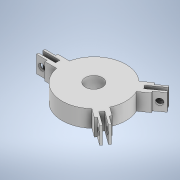
# Autodesk Inventor part: actuatorLink
Saved by Autodesk Inventor 2021 (Build 250183000, 183)
## iProperties
Created: 2020-12-19
Part Number: actuatorLink
Material: Generic
Document SubType Name: Modeling
Designer: awitc
Density: 1 g/cm^3
Appearance: Default
Author: awitc
Autodesk Inventor part; units mm, degrees
ref_plane "YZ Plane" through (0, 0, 0) normal (1, 0, 0) x (0, 1, 0)
ref_plane "XZ Plane" through (0, 0, 0) normal (0, 1, 0) x (-1, 0, 0)
ref_plane "XY Plane" through (0, 0, 0) normal (0, 0, 1) x (1, 0, 0)
sketch "Sketch1" plane through (0, 0, 0) normal (0, 1, 0) x (-1, 0, 0)
  circle A0 centre (-0.1978, 0.0875) radius 15
  line L0 (0, 0) -> (25, 0)
  line L1 (0, 0) -> (-20.2254, -14.6946)
  line L2 (0, 0) -> (25, 0) construction
  line L3 (0, 0) -> (-20.2254, 14.6946)
  line L4 (0, 0) -> (25, 0) construction
  line L5 (25, 0) -> (14.5167, 0)
  line L6 (25, 0) -> (14.481, 0)
  line L7 (25, 2) -> (20, 2)
  line L8 (20, 2) -> (20, -2)
  line L9 (20, -2) -> (25, -2)
  line L10 (20, -2) -> (20, -3)
  line L11 (20, 2) -> (20, 3)
  line L12 (25, -2) -> (25, 2)
  line L13 (20, 3) -> (14.5167, 3)
  line L14 (20, -3) -> (14.481, -3)
  line L15 (-21.401, 13.0766) -> (-17.3559, 10.1377)
  line L16 (-17.3559, 10.1377) -> (-17.9437, 9.3287)
  line L17 (-19.0499, 16.3127) -> (-15.0048, 13.3737)
  line L18 (-15.0048, 13.3737) -> (-14.417, 14.1828)
  line L19 (-19.0499, 16.3127) -> (-21.401, 13.0766)
  line L20 (-17.9437, 9.3287) -> (-13.832, 6.3413)
  line L21 (-14.417, 14.1828) -> (-10.2902, 11.1845)
  line L22 (-19.0499, -16.3127) -> (-15.0048, -13.3737)
  line L23 (-15.0048, -13.3737) -> (-14.417, -14.1828)
  line L24 (-17.9437, -9.3287) -> (-17.3559, -10.1377)
  line L25 (-17.3559, -10.1377) -> (-21.401, -13.0766)
  line L26 (-19.0499, -16.3127) -> (-21.401, -13.0766)
  line L27 (-14.417, -14.1828) -> (-10.1826, -11.1063)
  line L28 (-17.9437, -9.3287) -> (-13.7712, -6.2971)
  line L29 (-17.9437, -9.3287) -> (-12.7862, -9.3287) construction
  point P0 (22.9129, 10)
  point P1 (-9.5074, 11.849)
  point P2 (-14.229, 5.3909)
  point P3 (-14.2604, -5.1319)
  point P4 (-9.5775, -11.6181)
  point P5 (14.2709, 4.0444)
  point P6 (14.247, -3.9556)
  dimension "d87" = 25
  dimension "d88" = 25
  dimension "d89" = 144
  dimension "d90" = 25
  dimension "d91" = 144
  dimension "d146" = 5
  dimension "d147" = 4
  dimension "d149" = 5
  dimension "d151" = 5
  dimension "d153" = 5
  dimension "d154" = 1
  dimension "d155" = 36
  constraints: 60 end point, 5 horizontal, 4 perpendicular, 3 equal length, 2 parallel, 2 point on line, 1 vertical, 14 other
  measures "d87" distance of L0.start L0.end
  measures "d88" distance of L0.start L1.end
  measures "d89" angle of L1 L2
  measures "d90" distance of L0.start L3.end
  measures "d91" angle of L4 L3
  measures "d146" distance of L7.start L7.end
  measures "d147" distance of L7.end L8.end
  measures "d149" distance of L15.start L15.end
  measures "d151" distance of L17.start L17.end
  measures "d153" distance of L22.start L22.end
  measures "d154" distance of L24.start L24.end
  measures "d155" angle of L29 L28
extrude "Extrusion1" add sketch "Sketch1" along normal blind 8
sketch "Sketch8" plane through (0, 8, 0) normal (0, 1, 0) x (1, 0, 0)
  circle A0 centre (0, 0) radius 4
  dimension "d80" = 8
  constraints: 1 centre point
  measures "d80" diameter of A0
extrude "Extrusion8" cut sketch "Sketch8" against normal blind 10
sketch "Sketch28" plane through (19.0499, 0, -16.3127) normal (0.809, 0, -0.5878) x (-0.5878, 0, -0.809)
  line L0 (-4, 8) -> (0, 8) projected
  line L1 (-2, 8) -> (-2, 0)
  line L2 (-2, 0) -> (-1, 0)
  line L3 (-4, 0) -> (0, 0) projected
  line L4 (-1, 0) -> (-1, 8)
  line L5 (-1, 8) -> (-3, 8)
  line L6 (-3, 8) -> (-3, 0)
  line L7 (-3, 0) -> (-1, 0)
  point P0 (-3, 8)
  point P1 (-3, 0)
  point P2 (-1, 8)
  dimension "d156" = 1
  dimension "d157" = 2
  constraints: 12 end point, 3 perpendicular, 2 point on line, 1 collinear, 1 midpoint, 1 vertical
  measures "d156" distance of L1.end L2.end
  measures "d157" distance of L4.end L5.end
extrude "Extrusion26" cut sketch "Sketch28" against normal blind 8
sketch "Sketch29" plane through (21.401, 0, 13.0766) normal (0.809, 0, 0.5878) x (0.5878, 0, -0.809)
  line L0 (-4, 8) -> (0, 8) projected
  line L1 (-2, 0) -> (-1, 0)
  line L2 (-1, 0) -> (-1, 8)
  line L3 (-1, 8) -> (-2, 8)
  line L4 (-2, 8) -> (-2, 0)
  line L5 (-4, 0) -> (0, 0) projected
  line L6 (-1, 8) -> (-3, 8)
  line L7 (-3, 8) -> (-3, 0)
  line L8 (-3, 0) -> (-1, 0)
  line L9 (-1, 0) -> (-1, 8)
  point P0 (-3, 8)
  dimension "d160" = 1
  dimension "d161" = 2
  constraints: 16 end point, 4 parallel, 2 horizontal, 2 perpendicular, 2 point on line
  measures "d160" distance of L3.end L2.end
  measures "d161" distance of L8.end L7.end
extrude "Extrusion27" cut sketch "Sketch29" against normal blind 8
sketch "Sketch30" plane through (-25, 0, -2) normal (-1, 0, 0) x (0, 0, 1)
  line L0 (8.3413, 8) -> (-4.2971, 8) projected
  line L1 (2, 0) -> (3, 0)
  line L2 (3, 0) -> (3, 8)
  line L3 (3, 8) -> (2, 8)
  line L4 (2, 8) -> (2, 0)
  line L5 (8.3413, 0) -> (-4.2971, 0) projected
  line L6 (2, 8) -> (1, 8)
  line L7 (1, 8) -> (1, 0)
  line L8 (1, 0) -> (2, 0)
  line L9 (2, 0) -> (2, 8)
  dimension "d164" = 1
  dimension "d165" = 1
  constraints: 16 end point, 4 parallel, 2 horizontal, 2 perpendicular, 2 point on line
  measures "d164" distance of L3.end L2.end
  measures "d165" distance of L8.end L7.end
extrude "Extrusion28" cut sketch "Sketch30" against normal blind 8
sketch "Sketch31" plane through (-25, 0, 2) normal (0, 0, 1) x (1, 0, 0)
  line L0 (5, 8) -> (0, 8) projected
  line L1 (0, 8) -> (4.994, 0)
  line L2 (0, 0) -> (8, 0) projected
  circle A0 centre (2.497, 4) radius 1.5
  point P0 (25, 0)
  dimension "d168" = 3
  constraints: 2 end point, 1 centre point, 1 midpoint, 1 point on line
  measures "d168" diameter of A0
sketch "Sketch32" plane through (17.3559, 0, 10.1377) normal (0.5878, 0, -0.809) x (-0.809, 0, -0.5878)
  line L0 (-5, 0) -> (0, 0) projected
  line L1 (3, 8) -> (-5, 8) projected
  line L2 (0, 0) -> (-5, 8)
  circle A0 centre (-2.5, 4) radius 1.5
  point P0 (20, 0)
  dimension "d169" = 3
  constraints: 2 end point, 1 centre point, 1 midpoint
  measures "d169" diameter of A0
sketch "Sketch33" plane through (15.0048, 0, -13.3737) normal (-0.5878, 0, -0.809) x (-0.809, 0, 0.5878)
  line L0 (-5, 8) -> (0, 8) projected
  line L1 (0, 0) -> (0, 8) projected
  line L2 (-5, 8) -> (0, 0)
  circle A0 centre (-2.5, 4) radius 1.5
  point P0 (20, 0)
  dimension "d170" = 3
  constraints: 2 end point, 1 centre point, 1 midpoint
  measures "d170" diameter of A0
extrude "Extrusion29" cut sketch "Sketch33" against normal blind 8 contours A0 L2 | L2 A0
extrude "Extrusion30" cut sketch "Sketch32" against normal blind 8
extrude "Extrusion31" cut sketch "Sketch31" against normal blind 8
body "Solid1"
